TRANSFO (Autodesk Fusion 360 design; units mm, degrees)
Autodesk Fusion 360 part; units mm, degrees
sketch "Esquisse1" plane through (0, 0, 0) normal (0, 0, 1) x (1, 0, 0)
  line L0 (14.75, -26.95) -> (-14.75, -26.95)
  line L1 (-14.75, -26.95) -> (-14.75, 26.95)
  line L2 (-14.75, 26.95) -> (14.75, 26.95)
  line L3 (14.75, 26.95) -> (14.75, -26.95)
  line L4 (14.75, -26.95) -> (-14.75, 26.95) construction
  line L5 (-14.75, -26.95) -> (14.75, 26.95) construction
  dimension "d1" = 29.5
  dimension "d2" = 53.9
  constraint horizontal L0
  constraint perpendicular L0 L1
  constraint parallel L0 L2
  constraint parallel L1 L3
  constraint coincident L4 origin
  constraint coincident L5 origin
  measures "d1" distance of L1.end L2.end
  measures "d2" distance of L0.end L1.end
extrude "Extrusion1" add sketch "Esquisse1" along normal blind 34.15
sketch "Esquisse6" plane through (-14.75, 0, 0) normal (-1, 0, 0) x (0, -1, 0)
  line L0 (-26.95, 0) -> (26.95, 0)
  line L1 (26.95, 0) -> (26.95, 34.15)
  line L2 (26.95, 34.15) -> (-26.95, 34.15)
  line L3 (-26.95, 34.15) -> (-26.95, 0)
extrude "Extrusion5" add sketch "Esquisse6" along normal blind 25.5
fillet "Congé1" radius 17 2 edges at (-40.25, 0, 34.15) (-40.25, 0, 0)
sketch "Esquisse2" plane through (14.75, 0, 0) normal (1, 0, 0) x (0, 1, 0)
  line L0 (-26.95, 0) -> (26.95, 0)
  line L1 (26.95, 0) -> (26.95, 34.15)
  line L2 (26.95, 34.15) -> (-26.95, 34.15)
  line L3 (-26.95, 34.15) -> (-26.95, 0)
  line L4 (10.15, 2.8565) -> (-16.15, 2.8565)
  line L5 (-16.15, 2.8565) -> (-16.15, 8.1565)
  line L6 (-16.15, 8.1565) -> (10.15, 8.1565)
  line L7 (10.15, 8.1565) -> (10.15, 2.8565)
  line L8 (10.15, 2.8565) -> (-16.15, 8.1565) construction
  line L9 (-16.15, 2.8565) -> (10.15, 8.1565) construction
  point P0 (-3, 5.5065)
  dimension "d5" = 26.3
  dimension "d6" = 5.3
  dimension "d82" = 5.5065
  dimension "d83" = 3
  constraint horizontal L4
  constraint perpendicular L4 L5
  constraint parallel L4 L6
  constraint parallel L5 L7
  constraint coincident L8 P0
  constraint coincident L9 P0
  measures "d5" distance of L5.end L6.end
  measures "d6" distance of L4.end L5.end
  measures "d82" distance of L0 P0
  measures "d83" horizontal distance of origin P0
extrude "Extrusion2" add sketch "Esquisse2" along normal blind 9 contours L4 L5 L6 L7
sketch "Esquisse3" plane through (0, 0, 8.1565) normal (0, 0, 1) x (-1, 0, 0)
  line L0 (-14.75, -10.15) -> (-14.75, 16.15)
  line L1 (-14.75, 16.15) -> (-23.75, 16.15)
  line L2 (-23.75, 16.15) -> (-23.75, -10.15)
  line L3 (-23.75, -10.15) -> (-14.75, -10.15)
  circle A0 centre (-19.25, 11.35) radius 1.8
  circle A1 centre (-19.25, -5.35) radius 1.8
  line L4 (-19.25, -3.55) -> (-23.75, -3.55)
  line L5 (-19.25, -7.15) -> (-23.75, -7.15)
  dimension "d9" = 3.6
  dimension "d10" = 3.6
  dimension "d11" = 4.8
  dimension "d12" = 4.5
  dimension "d13" = 4.5
  dimension "d14" = 4.8
  constraint coincident A1 L4.start
  constraint coincident L2 L4.end
  constraint tangent A1 L4
  constraint perpendicular L2 L4
  constraint coincident A1 L5.start
  constraint coincident L2 L5.end
  constraint tangent A1 L5
  constraint perpendicular L2 L5
  measures "d9" diameter of A0
  measures "d10" diameter of A1
  measures "d11" distance of L1 A0.centre
  measures "d12" distance of L2 A0.centre
  measures "d13" distance of L2 A1.centre
  measures "d14" distance of L3 A1.centre
hole "Perçage1" at (19.25, -11.35, 8.1565) at (19.25, 5.35, 8.1565) direction (0, 0, -1) diameter 3.6 end through all
sketch "Esquisse4" plane through (14.75, 0, 0) normal (1, 0, 0) x (0, 1, 0)
  line L0 (10.15, 8.1565) -> (10.15, 2.8565)
  line L1 (10.15, 2.8565) -> (-16.15, 2.8565)
  line L2 (-16.15, 2.8565) -> (-16.15, 8.1565)
  line L3 (-16.15, 8.1565) -> (10.15, 8.1565)
  line L4 (-26.95, 0) -> (26.95, 0)
  line L5 (26.95, 0) -> (26.95, 34.15)
  line L6 (26.95, 34.15) -> (-26.95, 34.15)
  line L7 (-26.95, 34.15) -> (-26.95, 0)
  circle A0 centre (-17.45, 25.4) radius 4.05
  circle A1 centre (19.3, 26) radius 4.05
  dimension "d18" = 8.1
  dimension "d19" = 8.1
  dimension "d20" = 9.5
  dimension "d21" = 7.65
  dimension "d22" = 8.75
  dimension "d23" = 8.15
  measures "d18" diameter of A0
  measures "d19" diameter of A1
  measures "d20" distance of L7 A0.centre
  measures "d21" distance of L5 A1.centre
  measures "d22" distance of L6 A0.centre
  measures "d23" distance of L6 A1.centre
extrude "Extrusion3" add sketch "Esquisse4" along normal blind 15 contours A0 | A1
sketch "Esquisse5" plane through (0, 26.95, 0) normal (0, 1, 0) x (-1, 0, 0)
  line L0 (-14.75, 0) -> (23.25, 0)
  line L1 (23.25, 34.15) -> (-14.75, 34.15)
  line L2 (-14.75, 34.15) -> (-14.75, 0)
  line L3 (18.6, 24.125) -> (70.2, 24.125)
  line L4 (70.2, 24.125) -> (70.2, 10.025)
  line L5 (70.2, 10.025) -> (18.6, 10.025)
  line L6 (18.6, 10.025) -> (18.6, 24.125)
  arc A0 (23.25, 0) -> (40.25, 17) centre (23.25, 17) ccw
  line L7 (40.25, 17) -> (40.25, 17.15)
  arc A1 (40.25, 17.15) -> (23.25, 34.15) centre (23.25, 17.15) ccw
  dimension "d26" = 51.6
  dimension "d27" = 14.1
  dimension "d28" = 10.025
  dimension "d29" = 10.025
  constraint horizontal L3
  constraint vertical L4
  constraint horizontal L5
  constraint vertical L6
  measures "d26" distance of L3.start L3.end
  measures "d27" distance of L3.end L4.end
  measures "d28" distance of L0 L5
  measures "d29" distance of L1 L3
extrude "Extrusion4" add sketch "Esquisse5" along normal blind 7.5 and the other way blind 63.1 contours L3 L4 L5 A0 L7 A1 | L3 L5 L6 A0 L7 A1
sketch "Esquisse7" plane through (0, 0, 24.125) normal (0, 0, 1) x (-1, 0, 0)
  line L0 (38.7532, -26.95) -> (18.6, -26.95)
  line L1 (18.6, -26.95) -> (18.6, -34.45)
  line L2 (18.6, -34.45) -> (70.2, -34.45)
  line L3 (70.2, -34.45) -> (70.2, 36.15)
  line L4 (70.2, 36.15) -> (18.6, 36.15)
  line L5 (18.6, 36.15) -> (18.6, 26.95)
  line L6 (18.6, 26.95) -> (38.7532, 26.95)
  line L7 (38.7532, 26.95) -> (38.7532, -26.95)
  line L8 (70.2, 36.15) -> (44.3, 36.15)
  line L9 (44.3, 36.15) -> (44.3, -34.45)
  line L10 (44.3, -34.45) -> (70.2, -34.45)
  line L11 (70.2, -34.45) -> (70.2, 36.15)
  dimension "d38" = 25.9
  constraint horizontal L8
  constraint vertical L9
  constraint horizontal L10
  constraint vertical L11
  constraint coincident L2 L9.end
  constraint coincident L3.end L4.start
  measures "d38" distance of L3.end L8.end
extrude "Extrusion6" add sketch "Esquisse7" along normal blind 8 and the other way blind 21.9 contours L2 L3 L4 L8 L9 L10 L11
sketch "Esquisse8" plane through (0, 0, 2.225) normal (0, 0, -1) x (1, 0, 0)
  line L0 (-49.45, -18.65) -> (-68.55, -18.65)
  line L1 (-68.55, -18.65) -> (-68.55, 20.35)
  line L2 (-68.55, 20.35) -> (-49.45, 20.35)
  line L3 (-49.45, 20.35) -> (-49.45, -18.65)
  line L4 (-49.45, -18.65) -> (-68.55, 20.35) construction
  line L5 (-68.55, -18.65) -> (-49.45, 20.35) construction
  line L6 (-68.55, 20.35) -> (-64.55, 20.35)
  line L7 (-64.55, 20.35) -> (-64.55, 18.75)
  line L8 (-64.55, 18.75) -> (-68.55, 18.75)
  line L9 (-68.55, 18.75) -> (-68.55, 20.35)
  line L10 (-49.45, 20.35) -> (-53.45, 20.35)
  line L11 (-53.45, 20.35) -> (-53.45, 18.75)
  line L12 (-53.45, 18.75) -> (-49.45, 18.75)
  line L13 (-49.45, 18.75) -> (-49.45, 20.35)
  line L14 (-68.55, -18.65) -> (-64.55, -18.65)
  line L15 (-64.55, -18.65) -> (-64.55, -17.05)
  line L16 (-64.55, -17.05) -> (-68.55, -17.05)
  line L17 (-68.55, -17.05) -> (-68.55, -18.65)
  line L18 (-49.45, -18.65) -> (-53.45, -18.65)
  line L19 (-53.45, -18.65) -> (-53.45, -17.05)
  line L20 (-53.45, -17.05) -> (-49.45, -17.05)
  line L21 (-49.45, -17.05) -> (-49.45, -18.65)
  line L22 (-70.2, -34.45) -> (-44.3, -34.45)
  point P0 (-59, 0.85)
  dimension "d64" = 19.1
  dimension "d65" = 39
  dimension "d66" = 4
  dimension "d67" = 1.6
  dimension "d68" = 4
  dimension "d69" = 1.6
  dimension "d70" = 4
  dimension "d71" = 1.6
  dimension "d72" = 4
  dimension "d73" = 1.6
  dimension "d74" = 35.3
  constraint horizontal L0
  constraint perpendicular L0 L1
  constraint parallel L0 L2
  constraint parallel L1 L3
  constraint coincident L4 P0
  constraint coincident L5 P0
  constraint horizontal L6
  constraint vertical L7
  constraint horizontal L8
  constraint vertical L9
  constraint horizontal L10
  constraint vertical L11
  constraint horizontal L12
  constraint vertical L13
  constraint horizontal L14
  constraint vertical L15
  constraint horizontal L16
  constraint vertical L17
  constraint horizontal L18
  constraint vertical L19
  constraint horizontal L20
  constraint vertical L21
  measures "d64" distance of L1.end L2.end
  measures "d65" distance of L0.end L1.end
  measures "d66" distance of L1.end L6.end
  measures "d67" distance of L1.end L8.end
  measures "d68" distance of L2.end L10.end
  measures "d69" distance of L2.end L12.end
  measures "d70" distance of L0.end L14.end
  measures "d71" distance of L0.end L16.end
  measures "d72" distance of L0.start L18.end
  measures "d73" distance of L0.start L20.end
  measures "d74" distance of P0 L22
extrude "Extrusion7" add sketch "Esquisse8" along normal blind 6 contours L0 L3 L18 L19 L20 L21 | L0 L1 L14 L15 L16 L17 | L2 L3 L10 L11 L12 L13 | L1 L2 L6 L7 L8 L9
sketch "Esquisse9" plane through (14.75, 0, 0) normal (1, 0, 0) x (0, 1, 0)
  circle A0 centre (19.3, 26) radius 4.05
  circle A1 centre (-17.45, 25.4) radius 4.05
  line L0 (10.15, 8.1565) -> (10.15, 2.8565)
  line L1 (10.15, 2.8565) -> (-16.15, 2.8565)
  line L2 (-16.15, 2.8565) -> (-16.15, 8.1565)
  line L3 (-16.15, 8.1565) -> (10.15, 8.1565)
  line L4 (-26.95, 0) -> (26.95, 0)
  line L5 (26.95, 0) -> (26.95, 34.15)
  line L6 (26.95, 34.15) -> (-26.95, 34.15)
  line L7 (-26.95, 34.15) -> (-26.95, 0)
  line L8 (-26.95, 34.15) -> (26.95, 34.15)
  line L9 (26.95, 34.15) -> (26.95, 32.05)
  line L10 (26.95, 32.05) -> (-26.95, 32.05)
  line L11 (-26.95, 32.05) -> (-26.95, 34.15)
  line L12 (-26.95, 0) -> (26.95, 0)
  line L13 (26.95, 0) -> (26.95, 2.8565)
  line L14 (26.95, 2.8565) -> (-26.95, 2.8565)
  line L15 (-26.95, 2.8565) -> (-26.95, 0)
  dimension "d57" = 2.1
  constraint horizontal L8
  constraint vertical L9
  constraint horizontal L10
  constraint vertical L11
  constraint coincident L5 L9.end
  constraint coincident L6.end L7.start
  constraint horizontal L12
  constraint vertical L13
  constraint horizontal L14
  constraint vertical L15
  constraint coincident L5 L13.end
  constraint coincident L4.start L7.end
  measures "d57" distance of L6.end L10.end
extrude "Extrusion8" cut sketch "Esquisse9" against normal blind 14 contours L1 L4 L5 L7 L12 L13 L14 L15 | L5 L6 L7 L8 L9 L10 L11
equation "d1 = 37.2 mm - 3.85 * 2 mm"
equation "d20 = 13.55 mm - 4.05 mm"
equation "d21 = 11.7 mm - ( 8.1 / 2 ) * 1 mm"
equation "d22 = 10.7 mm - ( ( 8.1 / 2 ) * 1 ) * 1 mm + 2.1 mm"
equation "d23 = 10.1 mm - ( ( 8.1 / 2 ) * 1 ) * 1 mm + 2.1 mm"
equation "Transfo_notch_larg = 1.6 mm"
equation "Transfo_notch_long = 4 mm"
equation "Transfo_B2Notch_larg = 11.90 mm" comment "Distance entre deux encoches dans la largeur"
equation "Transfo_B2Notch_long = 39 mm - ( 2 * 1.6 ) * 1 mm" comment "Distance entre deux encoches dans la longueur"
equation "Transfo_hole_diam = 3.7 mm" comment "Diamètre du trou pour fixer le transfo"
equation "Transfo_hole_dist = 16.7 mm" comment "Distance entre les deux trous du transfo"
equation "Transfo_Dist_notch_hole = 69.2 mm" comment "Distance entre les trous (centre) et les encoches"
